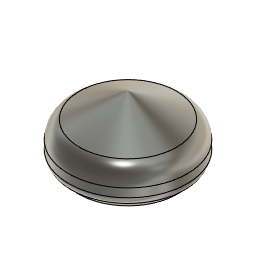
ORS_Button_Pin (Autodesk Fusion 360 design; units mm, degrees)
Autodesk Fusion 360 part; units mm, degrees
sketch "Main Body Sketch" plane through (0, 0, 0) normal (0, 0, 1) x (1, 0, 0)
  circle A0 centre (0, 0) radius 3
  dimension "d1" = 6
  constraint coincident A0.centre origin
  measures "d1" diameter of A0
extrude "Extrude1" add sketch "Main Body Sketch" along normal blind 1.75
sketch "Pin Point Sketch" plane through (0, 0, 0) normal (0, 1, 0) x (1, 0, 0)
  line L0 (-3, -1.75) -> (3, -1.75)
  line L1 (3, -1.75) -> (0, -3.29)
  line L2 (0, -3.29) -> (0, -1.75)
  dimension "d4" = 1.54
  constraint coincident L0.end L1.start
  constraint midpoint L0 L2.end
  constraint perpendicular L0 L2
  measures "d4" distance of L1.end L2.end
revolve "Revolve1" add sketch "Pin Point Sketch" angle 360 about axis through (0, 0, 0) along (0, 0, -1)
fillet "Fillet1" radius 1 1 edges at (-2.797, -1.0848, 1.75)
chamfer "Chamfer1" distance 0.5 angle 45 1 edges at (-2.797, -1.0848, 0)
fillet "Fillet2" radius 0.5 1 edges at (-2.797, 1.0848, 0.5)
named bodies: "ORS_Button_Pin"
